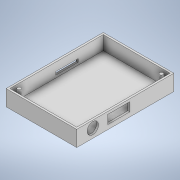
# Autodesk Inventor part: carcasaDisplayAdapter
Saved by Autodesk Inventor 2020 (Build 240168000, 168)
## iProperties
Created: 2021-04-22
Part Number: carcasaDisplayAdapter
Material: Generic
Document SubType Name: Modeling
Designer: Vlasciar
Density: 1 g/cm^3
Appearance: Default
Author: Vlasciar
Autodesk Inventor part; units mm, degrees
ref_plane "YZ Plane" through (0, 0, 0) normal (1, 0, 0) x (0, 1, 0)
ref_plane "XZ Plane" through (0, 0, 0) normal (0, 1, 0) x (-1, 0, 0)
ref_plane "XY Plane" through (0, 0, 0) normal (0, 0, 1) x (1, 0, 0)
sketch "Sketch1" plane through (0, 0, 0) normal (0, 1, 0) x (-1, 0, 0)
  line L0 (-28, -38.5) -> (28, -38.5)
  line L1 (28, -38.5) -> (28, 38.5)
  line L2 (28, 38.5) -> (-28, 38.5)
  line L3 (-28, 38.5) -> (-28, -38.5)
  line L4 (-28, -38.5) -> (28, 38.5) construction
  line L5 (28, -38.5) -> (-28, 38.5) construction
  point P0 (0, 0)
  dimension "d0" = 56
  dimension "d1" = 77
  constraints: 12 end point, 2 midpoint, 2 parallel, 1 horizontal, 1 perpendicular
  measures "d0" distance of L1.end L2.end
  measures "d1" distance of L0.end L1.end
extrude "Extrusion1" add sketch "Sketch1" along normal blind 12.5
shell "Shell1" thickness 1.5 removed faces 1 at (9.3333, 12.5, 12.8333)
sketch "Sketch2" plane through (28, 0, 38.5) normal (1, 0, 0) x (0, 0, -1)
  line L0 (0, 0) -> (77, 0) projected
  line L1 (0, 12.5) -> (77, 12.5) projected
  line L2 (15.5784, 3.5) -> (18, 3.5)
  circle A0 centre (12.75, 7) radius 4.5
  line L3 (1.5, 1.5) -> (1.5, 12.5) projected
  line L4 (42, 3.5) -> (24.5, 3.5)
  line L5 (24.5, 3.5) -> (24.5, 10.5)
  line L6 (24.5, 10.5) -> (42, 10.5)
  line L7 (42, 10.5) -> (42, 3.5)
  line L8 (42, 3.5) -> (24.5, 10.5) construction
  line L9 (24.5, 3.5) -> (42, 10.5) construction
  point P0 (38.5, 0)
  point P1 (33.25, 7)
  point P2 (33.25, 7)
  dimension "d10" = 9
  dimension "d7" = 3.5
  dimension "d8" = 3.5
  dimension "d9" = 5.5
  dimension "d11" = 6.75
  dimension "d12" = 17.5
  dimension "d13" = 7
  dimension "d14" = 23
  constraints: 14 end point, 3 midpoint, 2 horizontal, 2 parallel, 1 coincident, 1 horizontal alignment, 1 perpendicular, 3 other
  measures "d7" distance between parallel lines of L0 L2
  measures "d8" distance from line of L2 point (12.75, 7)
  measures "d9" distance from line of L1 point (12.75, 7)
  measures "d12" distance of L5.end L6.end
  measures "d13" distance of L6.end L4.start
  measures "d14" distance between parallel lines of L3 L5
extrude "Extrusion2" cut sketch "Sketch2" against normal blind 12.5
sketch "Sketch3" plane through (-28, 0, -38.5) normal (-1, 0, 0) x (0, 0, 1)
  line L0 (0, 0) -> (77, 0) projected
  line L1 (40, 3.5) -> (20.5, 3.5)
  line L2 (20.5, 3.5) -> (20.5, 6)
  line L3 (20.5, 6) -> (40, 6)
  line L4 (40, 6) -> (40, 3.5)
  line L5 (40, 3.5) -> (20.5, 6) construction
  line L6 (20.5, 3.5) -> (40, 6) construction
  line L7 (1.5, 1.5) -> (1.5, 12.5) projected
  line L8 (21.5, 6) -> (21.5, 3.5)
  line L9 (39, 6) -> (39, 3.4503)
  point P0 (38.5, 0)
  point P1 (30.25, 4.75)
  point P2 (39, 3.5)
  dimension "d17" = 3.5
  dimension "d18" = 2.5
  dimension "d19" = 19.5
  dimension "d20" = 19
  dimension "d21" = 1
  dimension "d22" = 1
  constraints: 16 end point, 2 midpoint, 2 parallel, 2 perpendicular, 2 point on line, 1 horizontal, 1 vertical
  measures "d17" distance between parallel lines of L0 L1
  measures "d18" distance of L3.end L1.start
  measures "d19" distance of L2.end L3.end
  measures "d20" distance between parallel lines of L7 L2
  measures "d21" distance between parallel lines of L8 L2
  measures "d22" distance between parallel lines of L4 L9
extrude "Extrusion3" cut sketch "Sketch3" against normal blind 12.5 contours L8 L3 L9 L1
sketch "Sketch4" plane through (-26.5, 1.5, -37) normal (0, 1, 0) x (1, 0, 0)
  line L0 (53, -74) -> (53, 0) projected
  line L1 (53, 0) -> (0, 0) projected
  line L2 (0, 0) -> (0, -74) projected
  line L3 (0, -74) -> (53, -74) projected
  circle A0 centre (3.725, -70.275) radius 1.375
  circle A1 centre (49.875, -3.825) radius 1.375
  point P0 (26.5, -37)
  dimension "d25" = 2.75
  dimension "d26" = 2.35
  dimension "d27" = 2.35
  dimension "d28" = 2.75
  dimension "d29" = 1.75
  dimension "d30" = 2.45
  constraints: 2 centre point
  measures "d25" diameter of A0
  measures "d26" distance edge to line of A0 L2
  measures "d27" distance edge to line of A0 L3
  measures "d28" diameter of A1
  measures "d29" distance edge to line of A1 L0
  measures "d30" distance edge to line of A1 L1
extrude "Extrusion4" add sketch "Sketch4" along normal blind 11 contours A0 | A1
body "Solid1"
